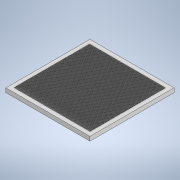
# Autodesk Inventor part: rendering_cmos_chip
Saved by Autodesk Inventor 2021 (Build 250183000, 183)
## iProperties
Created: 2021-06-18
Part Number: rendering_cmos_chip
Material: Generic
Document SubType Name: Modeling
Designer: MicroscopyInnovation
Density: 1 g/cm^3
Appearance: Default
Author: MicroscopyInnovation
Autodesk Inventor part; units mm, degrees
ref_plane "YZ Plane" through (0, 0, 0) normal (1, 0, 0) x (0, 1, 0)
ref_plane "XZ Plane" through (0, 0, 0) normal (0, 1, 0) x (-1, 0, 0)
ref_plane "XY Plane" through (0, 0, 0) normal (0, 0, 1) x (1, 0, 0)
sketch "Sketch1" plane through (0, 0, 0) normal (0, 1, 0) x (-1, 0, 0)
  line L0 (0, 0) -> (200, 0)
  line L1 (200, 0) -> (200, -200)
  line L2 (200, -200) -> (0, -200)
  line L3 (0, -200) -> (0, 0)
  dimension "d0" = 200
  dimension "d1" = 200
  constraints: 8 end point, 2 parallel, 1 horizontal, 1 perpendicular
  measures "d0" distance of L1.end L2.end
  measures "d1" distance of L0.end L1.end
extrude "Extrusion1" add sketch "Sketch1" along normal blind 10
sketch "Sketch2" plane through (0, 10, 0) normal (0, 1, 0) x (1, 0, 0)
  line L0 (-190, 10) -> (-10, 10)
  line L1 (-10, 10) -> (-10, 11)
  line L2 (-10, 11) -> (-190, 11)
  line L3 (-190, 11) -> (-190, 10)
  point P0 (0, 0)
  dimension "d4" = 180
  dimension "d5" = 1
  constraints: 8 end point, 2 parallel, 1 horizontal, 1 perpendicular
  measures "d4" distance of L2.end L1.end
  measures "d5" distance of L1.end L0.end
extrude "Extrusion2" add sketch "Sketch2" along normal blind 1
pattern_linear "Rectangular Pattern1" count 90 spacing 2 along (0, 0, -1) of "Extrusion2"
body "Solid1"
